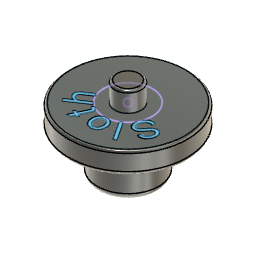
De Blokko v3 (Autodesk Fusion 360 design; units mm, degrees)
Autodesk Fusion 360 part; units mm, degrees
sketch "Sketch1" plane through (0, 0, 0) normal (1, 0, 0) x (0, 1, 0)
  line L0 (4, 0) -> (5.5, 0)
  line L1 (7, 1.5) -> (7, 8.537)
  line L2 (7.4617, 9.0355) -> (12.5576, 9.4275)
  line L3 (13.4809, 10.4246) -> (13.4809, 13.9985)
  line L4 (12.9809, 14.4985) -> (3, 14.4985)
  line L5 (0, 14.4985) -> (0, 10)
  arc A0 (7.4617, 9.0355) -> (7, 8.537) centre (7.5, 8.537) ccw
  arc A1 (12.5576, 9.4275) -> (13.4809, 10.4246) centre (12.4809, 10.4246) ccw
  arc A2 (5.5, 0) -> (7, 1.5) centre (5.5, 1.5) ccw
  arc A3 (13.4809, 13.9985) -> (12.9809, 14.4985) centre (12.9809, 13.9985) ccw
  line L6 (3, 14.4985) -> (3, 18.4985)
  line L7 (2.5, 18.9985) -> (0, 18.9985)
  line L8 (0, 18.9985) -> (0, 14.4985)
  arc A4 (3, 18.4985) -> (2.5, 18.9985) centre (2.5, 18.4985) ccw
  line L9 (4, 0) -> (4, 10)
  line L10 (4, 10) -> (0, 10)
  point P0 (7, 0)
  point P1 (7, 9)
  point P2 (13.4809, 9.4985)
  point P3 (13.4809, 14.4985)
  point P4 (3, 18.9985)
  dimension "d3" = 7
  dimension "d4" = 9
  dimension "d6" = 6.5
  dimension "d8" = 5
  dimension "d9" = 0.5
  dimension "d10" = 1
  dimension "d11" = 1.5
  dimension "d12" = 0.5
  dimension "d13" = 3
  dimension "d14" = 4.5
  dimension "d15" = 0.5
  dimension "d16" = 4
  dimension "d17" = 10
  dimension "d23" = 8.9985
  dimension "d24" = 4
  dimension "d25" = 9.9809
  dimension "d26" = 2.5
  dimension "d27" = 7.037
  dimension "d28" = 5.0959
  dimension "d29" = 3.574
  dimension "d30" = 4.4985
  dimension "d31" = 18.9985
  constraint horizontal L0
  constraint perpendicular L0 L1
  constraint vertical L3
  constraint perpendicular L3 L4
  constraint perpendicular L0 L5
  constraint coincident P1 L2
  constraint coincident P1 L1
  constraint tangent L2 A0
  constraint tangent L1 A0
  constraint coincident P2 L2
  constraint coincident P2 L3
  constraint tangent L2 A1
  constraint tangent L3 A1
  constraint coincident P0 L0
  constraint coincident P0 L1
  constraint tangent L0 A2
  constraint tangent L1 A2
  constraint coincident P3 L3
  constraint coincident P3 L4
  constraint tangent L3 A3
  constraint tangent L4 A3
  constraint perpendicular L6 L7
  constraint coincident P4 L7
  constraint coincident P4 L6
  constraint tangent L7 A4
  constraint tangent L6 A4
  constraint perpendicular L0 L9
  constraint perpendicular L5 L10
  measures "d3" distance of origin P0
  measures "d4" distance of P0 P1
  measures "d6" distance of P1 P2
  measures "d8" distance of P2 P3
  measures "d9" radius of A0
  measures "d10" radius of A1
  measures "d11" radius of A2
  measures "d12" radius of A3
  measures "d13" distance of L5.start L4.end
  measures "d14" distance of L4.end P4
  measures "d15" radius of A4
  measures "d16" distance of origin L0.start
  measures "d17" distance of L0.start L9.end
  measures "d23" distance of L7.end L5.end
  measures "d24" distance of L9.end L5.end
  measures "d25" distance of L4.start L4.end
  measures "d26" distance of L7.end L7.start
  measures "d27" distance of L1.end L1.start
  measures "d28" horizontal distance of L2.start L2.end
  measures "d29" distance of L3.start L3.end
  measures "d30" distance of L5.start L5.end
  measures "d31" distance of L0 L7
revolve "Revolve1" add sketch "Sketch1" angle 360 about axis through (0, 0, 14.4985) along (0, 0, -1)
sketch "Sketch3" plane through (0, 0, 14.4985) normal (0, 0, 1) x (-1, 0, 0)
  circle A0 centre (0, 0) radius 3
  circle A1 centre (0, 0) radius 12.9809
  circle A2 centre (0, 0) radius 5.5
  dimension "d20" = 5
  text T0 "Sloth " font "Arial" height 5 align left spacing 1 along the path A2 letters at x, y, angle (-11.736, 2.7356, 65.733) (-7.1535, 9.4457, 33.3828) (-2.9787, 11.6057, 5.0654) (4.1711, 11.1056, -25.2773) (8.6611, 8.2794, -55.62) (11.7257, 1.8004, -85.9626)
extrude "Extrude1" cut sketch "Sketch3" against normal blind 0.5 text T0
